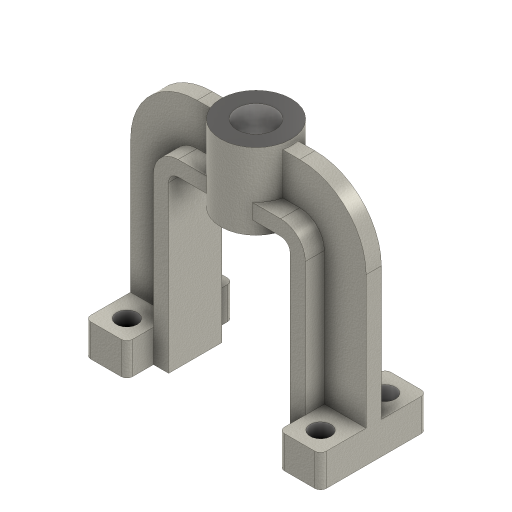
# Autodesk Inventor part: Part029. Shaft guide
Saved by Autodesk Inventor 2023.2 (Build 272271030, 271C)
## iProperties
Created: 2023-10-10
Part Number: Part029. Shaft guide
Material: Steel, Cast
Document SubType Name: Modeling
Designer: User
Mass: 1228.95 g
Surface Area: 446.59 cm^2
Volume: 156.555 cm^3
Density: 7.85 g/cm^3
Appearance: Steel - Cast
Author: User
Autodesk Inventor part; units mm, degrees
ref_plane "YZ Plane" through (0, 0, 0) normal (1, 0, 0) x (0, 1, 0)
ref_plane "XY Plane" through (0, 0, 0) normal (0, 0, 1) x (1, 0, 0)
sketch "Sketch1" plane through (0, 0, 0) normal (0, 0, 1) x (1, 0, 0)
  line L0 (-62, 0) -> (-62, 87)
  arc A0 (-27, 122) -> (-62, 87) centre (-27, 87) ccw
  line L1 (-27, 122) -> (27, 122)
  arc A1 (62, 87) -> (27, 122) centre (27, 87) ccw
  line L2 (62, 87) -> (62, 0)
  point P0 (0, 0)
  point P1 (0, 122)
  point P2 (62, 43.5)
  dimension "d0" = 122
  dimension "d1" = 124
  dimension "d2" = 35
  constraints: 6 end point, 4 point on circle, 4 tangent, 3 horizontal alignment, 2 centre point, 2 midpoint, 2 perpendicular, 1 equal radius, 1 vertical, 1 vertical alignment
  measures "d0" distance from line of L0.start L1
  measures "d1" distance from line of point (62, 43.5) L0
  measures "d2" radius of A0
sketch "Sketch2" plane through (0, 0, 0) normal (0, 1, 0) x (-1, 0, 0)
  line L0 (62, 4) -> (62, -4)
  line L1 (62, -4) -> (40, -4)
  line L2 (40, -4) -> (40, -14)
  line L3 (40, -14) -> (32, -14)
  line L4 (32, -14) -> (32, 14)
  line L5 (32, 14) -> (40, 14)
  line L6 (40, 14) -> (40, 4)
  line L7 (40, 4) -> (62, 4)
  point P0 (0, 0)
  point P1 (62, 0)
  point P2 (32, 0)
  point P3 (62, 0)
  dimension "d4" = 30
  dimension "d5" = 28
  dimension "d6" = 8
  dimension "d7" = 8
  constraints: 16 end point, 7 perpendicular, 2 midpoint, 1 coincident, 1 horizontal alignment, 1 parallel, 1 vertical
  measures "d4" distance between parallel lines of L4 L0
  measures "d5" distance between parallel lines of L3 L5
  measures "d6" distance between parallel lines of L4 L2
  measures "d7" distance between parallel lines of L1 L7
sweep "Sweep1" add profiles "Sketch2" path "Sketch1"
sketch "Sketch3" plane through (0, 0, 0) normal (0, 1, 0) x (-1, 0, 0)
  line L0 (-40, -28) -> (-62, -28)
  line L1 (-62, -28) -> (-62, 28)
  line L2 (-62, 28) -> (-40, 28)
  line L3 (-40, 28) -> (-40, -28)
  line L4 (-62, -4) -> (-62, 4) projected
  point P0 (0, 0)
  point P1 (-62, 0)
  dimension "d10" = 22
  dimension "d11" = 56
  constraints: 8 end point, 2 midpoint, 2 parallel, 1 horizontal, 1 perpendicular
  measures "d10" distance of L1.end L2.end
  measures "d11" distance of L0.end L1.end
extrude "Extrusion1" add sketch "Sketch3" along normal blind 17
fillet "Fillet1" radius 3 4 edges at (62, 8.5, 28) (40, 8.5, 28) (62, 8.5, -28) (40, 8.5, -28)
sketch "Sketch4" plane through (0, 17, 0) normal (0, 1, 0) x (1, 0, 0)
  line L0 (43, -28) -> (59, -28) projected
  line L1 (51, 17) -> (51, -17) construction
  point P0 (0, 0)
  point P1 (51, 0)
  point P2 (51, -28)
  dimension "d15" = 34
  constraints: 2 end point, 2 midpoint, 2 vertical alignment, 1 horizontal alignment
  measures "d15" distance of L1.end L1.start
hole "Hole1" at (51, 17, -17) at (51, 17, 17) direction (0, -1, 0) diameter 11 end through all
mirror "Mirror1" about plane through (0, 0, 0) normal (1, 0, 0) of "Extrusion1", "Fillet1", "Hole1"
ref_plane "Work Plane1" through (0, 125, 0) normal (0, 1, 0) x (-1, 0, 0)
sketch "Sketch5" plane through (0, 125, 0) normal (0, 1, 0) x (-1, 0, 0)
  circle A0 centre (0, 0) radius 18.5
  dimension "d24" = 37
  constraints: 1 centre point, 1 coincident
  measures "d24" diameter of A0
extrude "Extrusion2" add sketch "Sketch5" against normal blind 40
sketch "Sketch6" plane through (0, 125, 0) normal (0, 1, 0) x (1, 0, 0)
  circle A0 centre (0, 0) radius 18.5 projected
hole "Hole2" at (0, 125, 0) direction (0, -1, 0) diameter 20 end through all
body "Solid1"
